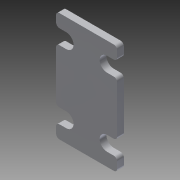
# Autodesk Inventor part: Aluminum Plate (0.125)
Saved by Autodesk Inventor 2014 (Build 180170000, 170)
## iProperties
Created: 2014-01-18
Part Number: Aluminum Plate (0.125)
Material: Aluminum 6061
Document SubType Name: Modeling
Designer: Andrew Toennies
Density: 2.71 g/cm^3
Appearance: Aluminum - Flat
Mass: 10.7618 g
Surface Area: 31.5253 cm^2
Volume: 3.97116 cm^3
Author: Andrew Toennies
Autodesk Inventor part; units mm, degrees
ref_plane "YZ Plane" through (0, 0, 0) normal (1, 0, 0) x (0, 1, 0)
ref_plane "XZ Plane" through (0, 0, 0) normal (0, 1, 0) x (-1, 0, 0)
ref_plane "XY Plane" through (0, 0, 0) normal (0, 0, 1) x (1, 0, 0)
sketch "Sketch1" plane through (0, 0, 0) normal (0, 0, 1) x (1, 0, 0)
  line L0 (1.5875, 0) -> (26.9875, 0)
  line L1 (26.9875, 51.1556) -> (1.5875, 51.1556)
  arc A0 (23.8125, 45.0215) -> (23.8125, 38.1635) centre (23.8125, 41.5925) ccw
  arc A1 (4.7625, 38.1635) -> (4.7625, 45.0215) centre (4.7625, 41.5925) ccw
  arc A2 (23.8125, 12.9921) -> (23.8125, 6.1341) centre (23.8125, 9.5631) ccw
  arc A3 (4.7625, 6.1341) -> (4.7625, 12.9921) centre (4.7625, 9.5631) ccw
  line L2 (4.7625, 41.5925) -> (23.8125, 41.5925) construction
  line L3 (23.8125, 9.5631) -> (23.8125, 41.5925) construction
  line L4 (4.7625, 41.5925) -> (4.7625, 9.5631) construction
  line L5 (4.7625, 9.5631) -> (23.8125, 9.5631) construction
  line L6 (4.7625, 6.1341) -> (1.5875, 6.1341)
  line L7 (4.7625, 12.9921) -> (1.5875, 12.9921)
  line L8 (23.8125, 12.9921) -> (26.9875, 12.9921)
  line L9 (23.8125, 6.1341) -> (26.9875, 6.1341)
  line L10 (23.8125, 38.1635) -> (26.9875, 38.1635)
  line L11 (23.8125, 45.0215) -> (26.9875, 45.0215)
  line L12 (4.7625, 45.0215) -> (1.5875, 45.0215)
  line L13 (4.7625, 38.1635) -> (1.5875, 38.1635)
  line L14 (0, 49.5681) -> (0, 46.609)
  line L15 (0, 36.576) -> (0, 14.5796)
  line L16 (0, 4.5466) -> (0, 1.5875)
  line L17 (28.575, 1.5875) -> (28.575, 4.5466)
  line L18 (28.575, 14.5796) -> (28.575, 36.576)
  line L19 (28.575, 46.609) -> (28.575, 49.5681)
  arc A4 (1.5875, 51.1556) -> (0, 49.5681) centre (1.5875, 49.5681) ccw
  arc A5 (28.575, 49.5681) -> (26.9875, 51.1556) centre (26.9875, 49.5681) ccw
  arc A6 (0, 1.5875) -> (1.5875, 0) centre (1.5875, 1.5875) ccw
  arc A7 (28.575, 4.5466) -> (26.9875, 6.1341) centre (26.9875, 4.5466) ccw
  arc A8 (26.9875, 0) -> (28.575, 1.5875) centre (26.9875, 1.5875) ccw
  arc A9 (26.9875, 12.9921) -> (28.575, 14.5796) centre (26.9875, 14.5796) ccw
  arc A10 (0, 14.5796) -> (1.5875, 12.9921) centre (1.5875, 14.5796) ccw
  arc A11 (1.5875, 6.1341) -> (0, 4.5466) centre (1.5875, 4.5466) ccw
  arc A12 (0, 46.609) -> (1.5875, 45.0215) centre (1.5875, 46.609) ccw
  arc A13 (1.5875, 38.1635) -> (0, 36.576) centre (1.5875, 36.576) ccw
  arc A14 (26.9875, 45.0215) -> (28.575, 46.609) centre (26.9875, 46.609) ccw
  arc A15 (28.575, 36.576) -> (26.9875, 38.1635) centre (26.9875, 36.576) ccw
  point P0 (0, 0)
  point P1 (28.575, 51.1556)
  point P2 (28.575, 0)
  point P3 (0, 51.1556)
  dimension "d0" = 28.575
  dimension "d1" = 51.1556
  dimension "d4" = 9.5631
  dimension "d5" = 9.5631
  dimension "d6" = 6.858
  dimension "d7" = 6.858
  dimension "d8" = 6.858
  dimension "d9" = 6.858
  dimension "d10" = 4.7625
  dimension "d11" = 4.7625
  dimension "d12" = 1.5875
  constraints: 40 end point, 32 point on circle, 32 tangent, 20 perpendicular, 16 centre point, 14 parallel, 12 point on line, 11 equal radius, 5 collinear, 1 horizontal
  measures "d0" distance of point (28.575, 51.156) point (0, 51.156)
  measures "d1" distance of point (28.575, 0) point (28.575, 51.156)
  measures "d4" distance between parallel lines of L0 L5
  measures "d5" distance between parallel lines of L1 L2
  measures "d6" diameter of A1
  measures "d7" diameter of A0
  measures "d8" diameter of A2
  measures "d9" diameter of A3
  measures "d10" distance between parallel lines of L3 L18
  measures "d11" distance between parallel lines of L15 L4
  measures "d12" radius of A4
extrude "Extrusion1" add sketch "Sketch1" along normal blind 3.175
body "Solid1"
